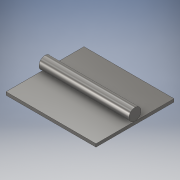
# Autodesk Inventor part: hinge
Saved by Autodesk Inventor 2019 (Build 230136000, 136)
## iProperties
Created: 2019-02-16
Part Number: hinge
Material: Stainless Steel
Document SubType Name: Modeling
Designer: suchanek
Density: 8 g/cm^3
Appearance: Semi-Polished
Author: suchanek
Autodesk Inventor part; units mm, degrees
ref_plane "YZ Plane" through (0, 0, 0) normal (1, 0, 0) x (0, 1, 0)
ref_plane "XZ Plane" through (0, 0, 0) normal (0, 1, 0) x (-1, 0, 0)
ref_plane "XY Plane" through (0, 0, 0) normal (0, 0, 1) x (1, 0, 0)
sketch "Sketch1" plane through (0, 0, 0) normal (1, 0, 0) x (0, 1, 0)
  line L0 (-0.25, 6.5) -> (0.25, 6.5)
  line L1 (0.25, 6.5) -> (0.25, -6.5)
  line L2 (0.25, -6.5) -> (-0.25, -6.5)
  line L3 (-0.25, -6.5) -> (-0.25, 6.5)
  line L4 (-0.25, 6.5) -> (0.25, -6.5) construction
  line L5 (0.25, 6.5) -> (-0.25, -6.5) construction
  circle A0 centre (1.25, 0) radius 1
  point P0 (0, 0)
  point P1 (0, 0)
  dimension "d0" = 0.5
  dimension "d1" = 13
  dimension "d2" = 2
  constraints: 12 end point, 3 midpoint, 2 parallel, 1 centre point, 1 horizontal, 1 horizontal alignment, 1 perpendicular, 1 tangent
  measures "d0" distance of L1.end L2.end
  measures "d1" distance of L0.end L1.end
  measures "d2" diameter of A0
extrude "Extrusion1" add sketch "Sketch1" along normal blind 15
body "Solid1"
